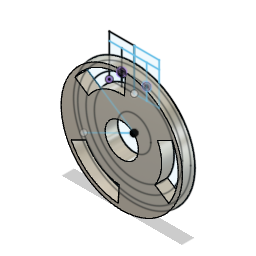
Universal encoder v6 (Autodesk Fusion 360 design; units mm, degrees)
Autodesk Fusion 360 part; units mm, degrees
sketch "Sketch17" plane through (0, 0, 0) normal (0, 0, 1) x (1, 0, 0)
  line L0 (0, 0) -> (0, 10)
  line L1 (0, 10) -> (6, 10)
  line L2 (6, 10) -> (6, 0)
  line L3 (6, 0) -> (0, 0)
  line L4 (0, 8) -> (6, 8)
  line L5 (3, 8) -> (3, 0)
  line L6 (3, 0) -> (3, 3)
  circle A0 centre (3, 3) radius 1
  line L7 (12, 10) -> (12, 0)
  line L8 (9, 0) -> (9, 3)
  line L9 (9, 8) -> (9, 0)
  line L10 (6, 8) -> (12, 8)
  circle A1 centre (9, 3) radius 1
  line L11 (12, 0) -> (6, 0)
  line L12 (6, 0) -> (6, 10)
  line L13 (6, 10) -> (12, 10)
  dimension "d299" = 10
  dimension "d300" = 6
  dimension "d301" = 3
  dimension "d302" = 2
  dimension "d308" = 10
  dimension "d309" = 6
  dimension "d310" = 3
  dimension "d311" = 2
  dimension "d333" = 6
  constraint coincident L0.start L3.end
  constraint vertical L0
  constraint perpendicular L0 L1
  constraint perpendicular L1 L2
  constraint perpendicular L0 L3
  constraint coincident L0 L4.start
  constraint coincident L2 L4.end
  constraint perpendicular L2 L4
  constraint midpoint L4 L5.start
  constraint midpoint L3 L5.end
  constraint coincident L5 L6.end
  constraint coincident L6.end A0.centre
  constraint vertical L12
  constraint perpendicular L12 L13
  constraint perpendicular L7 L13
  constraint perpendicular L11 L12
  constraint coincident L4.end L12
  constraint coincident L10.end L7
  constraint perpendicular L7 L10
  constraint midpoint L9.start L10
  constraint midpoint L8.start L11
  constraint coincident L8.end L9
  constraint coincident L8.end A1.centre
  measures "d299" distance of L0.start L0.end
  measures "d300" distance of L0.end L1.end
  measures "d301" distance of L5.end L6.end
  measures "d302" diameter of A0
  measures "d308" distance of L1.end L2.end
  measures "d309" distance of L1.end L7.start
  measures "d310" distance of L8.end L8.start
  measures "d311" diameter of A1
  measures "d333" distance of L6.end L8.end
sketch "Sketch18" plane through (0, 0, 0) normal (0, 0, 1) x (1, 0, 0)
  circle A0 centre (6, -8.1962) radius 11.5911
  circle A1 centre (6, -8.1962) radius 13.5911
  circle A2 centre (6, -8.1962) radius 9.5911
  line L0 (6, -8.1962) -> (-5.3131, -0.664)
  circle A3 centre (6, -8.1962) radius 14.5911
  line L1 (6, -8.1962) -> (-6.1795, -14.2275)
  circle A4 centre (6, -8.1962) radius 4
  point P0 (3, 3)
  point P1 (9, 3)
  point P2 (3, 3)
  point P3 (3, 3)
  point P4 (9, 3)
  point P5 (3, 3)
  dimension "d337" = 23.1822
  dimension "d339" = 11.5911
  dimension "d340" = 11.5911
  dimension "d341" = 27.1822
  dimension "d342" = 19.1822
  dimension "d347" = 29.1822
  dimension "d351" = 60
  dimension "d352" = 8
  constraint concentric A0 A1
  constraint concentric A0 A2
  constraint coincident A0.centre A1.centre
  constraint coincident A1 L0.end
  constraint concentric A2 A3
  measures "d337" diameter of A0
  measures "d339" distance of A0.centre P1
  measures "d340" distance of A0.centre P5
  measures "d341" diameter of A1
  measures "d342" diameter of A2
  measures "d347" diameter of A3
  measures "d352" diameter of A4
extrude "Extrude45" add sketch "Sketch18" along normal blind 3 contours A0 A2 L0 L1 | A0 A1 L0 L1 picked at (-3.6109, -3.0615) picked at (-5.0902, -1.6236) makes body 1
pattern_circular "C-Pattern13" count 3 over 360 about axis through (6, -8.1962, 0) along (0, 0, 1) of bodies 1 makes body 2 at (9.9587, -19.7633, 0) makes body 3 at (15.3213, -0.2851, 0)
extrude "Extrude46" add sketch "Sketch18" along normal blind 3 contours A2 L0 L1 A4 | A2 L0 L1 A4 | A3 bodies 1 2 3
equation "Enkoder_Kanal_Yüksekliği = 4 mm"
equation "Enkoder_Kanal_Sayısı = 3"
equation "Enkoder_Kanal_Çarpanı = 0"
equation "Enkoder_Sensör_Aralığı = 6 mm"
equation "milçapı = 8 mm"
equation "Enkoder_Kalınlığı = 3 mm"
equation "d333 = sensörAralığı"
equation "d337 = Enkoder_Sensör_Aralığı / 2 / ( sin(( ( 360 / Enkoder_Kanal_Sayısı / 2 * ( 2 * Enkoder_Kanal_Çarpanı + 1 ) / 2 ) / 2 ) * 1 deg) ) * 2"
equation "d339 = Enkoder_Sensör_Aralığı / 2 / ( sin(( ( 360 / Enkoder_Kanal_Sayısı / 2 * ( 2 * Enkoder_Kanal_Çarpanı + 1 ) / 2 ) / 2 ) * 1 deg) )"
equation "d340 = Enkoder_Sensör_Aralığı / 2 / ( sin(( ( 360 / Enkoder_Kanal_Sayısı / 2 * ( 2 * Enkoder_Kanal_Çarpanı + 1 ) / 2 ) / 2 ) * 1 deg) )"
equation "d341 = Enkoder_Sensör_Aralığı / 2 / ( sin(( ( 360 / Enkoder_Kanal_Sayısı / 2 * ( 2 * Enkoder_Kanal_Çarpanı + 1 ) / 2 ) / 2 ) * 1 deg) ) * 2 + Enkoder_Kanal_Yüksekliği"
equation "d342 = Enkoder_Sensör_Aralığı / 2 / ( sin(( ( 360 / Enkoder_Kanal_Sayısı / 2 * ( 2 * Enkoder_Kanal_Çarpanı + 1 ) / 2 ) / 2 ) * 1 deg) ) * 2 - Enkoder_Kanal_Yüksekliği"
equation "d343 = Enkoder_Kalınlığı"
equation "d345 = Enkoder_Kanal_Sayısı"
equation "d347 = Enkoder_Sensör_Aralığı / 2 / ( sin(( ( 360 / Enkoder_Kanal_Sayısı / 2 * ( 2 * Enkoder_Kanal_Çarpanı + 1 ) / 2 ) / 2 ) * 1 deg) ) * 2 + Enkoder_Kanal_Yüksekliği + 2 mm"
equation "d348 = Enkoder_Kalınlığı"
equation "d351 = ( 360 / Enkoder_Kanal_Sayısı / 2 ) * 1 deg"
equation "d352 = milçapı"
